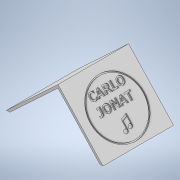
# Autodesk Inventor part: Tableros
Saved by Autodesk Inventor 2022.5 (Build 265521000, 521)
## iProperties
Created: 2023-09-03
Part Number: Tableros
Material: Genérico
Document SubType Name: Modeling
Designer: Carlos_Caucali
Density: 1 g/cm^3
Appearance: Valor por defecto
Author: Carlos_Caucali
Autodesk Inventor part; units mm, degrees
ref_plane "YZ Plane" through (0, 0, 0) normal (1, 0, 0) x (0, 1, 0)
ref_plane "XZ Plane" through (0, 0, 0) normal (0, 1, 0) x (-1, 0, 0)
ref_plane "XY Plane" through (0, 0, 0) normal (0, 0, 1) x (1, 0, 0)
sketch "Boceto1" plane through (0, 0, 0) normal (0, 0, 1) x (1, 0, 0)
  line L0 (0, 204.6955) -> (191.0491, 0) construction
  line L1 (191.0491, 0) -> (183.7386, -6.8232) construction
  line L2 (183.7386, -6.8232) -> (-7.3106, 197.8723) construction
  line L3 (-7.3106, 197.8723) -> (0, 204.6955)
  line L4 (0, 204.6955) -> (-219.3166, 0) construction
  line L5 (-219.3166, 0) -> (-212.4934, -7.3106) construction
  line L6 (-212.4934, -7.3106) -> (6.8232, 197.3849) construction
  line L7 (6.8232, 197.3849) -> (0, 204.6955)
  line L8 (0, 0) -> (0, 350) construction
  line L9 (-300, 0) -> (300, 0) construction
  line L10 (6.8232, 197.3849) -> (191.0491, 0)
  line L11 (177.3703, 0) -> (191.0491, 0)
  line L12 (0, 191.0166) -> (177.3703, 0)
  arc A0 (0, 191.0166) -> (-204.6607, 0) centre (37241.4186, -39915.6513) ccw
  line L13 (-204.6607, 0) -> (-219.3166, 0)
  line L14 (-204.6607, 0) -> (-219.3166, 0)
  line L15 (-219.3166, 0) -> (-7.3106, 197.8723)
  dimension "d0" = 280
  dimension "d1" = 300
  dimension "d2" = 10
  dimension "d3" = 10
  dimension "d4" = 350
  dimension "d5" = 600
  dimension "d6" = 0
  constraints: 30 end point, 7 point on line, 4 parallel, 2 horizontal, 2 perpendicular, 2 point on circle, 1 centre point, 1 collinear, 1 vertical, 10 other
  measures "d0" distance between parallel lines of L1 L4
  measures "d1" distance between parallel lines of L0 L5
  measures "d2" distance between parallel lines of L0 L2
  measures "d3" distance between parallel lines of L6 L4
  measures "d4" distance of L8.start L8.end
  measures "d5" distance of point (-300, 0) point (300, 0)
  measures "d6" distance of L8.start point (0, 0)
extrude "Extrusión1" add sketch "Boceto1" along normal mid plane 300
sketch "Boceto2" plane through (0, 204.6955, 150) normal (0.7310553, 0.6823183, 0) x (0, 0, -1)
  line L0 (300, 0) -> (0, 0) construction
  line L1 (0, -280) -> (0, 0) construction
  line L2 (300, -280) -> (0, -280) construction
  line L3 (300, 0) -> (300, -280) construction
  line L4 (60, -69.6437) -> (240, -69.6437) construction
  line L5 (240, -69.6437) -> (240, -229.6437) construction
  line L6 (240, -229.6437) -> (60, -229.6437) construction
  line L7 (60, -229.6437) -> (60, -69.6437) construction
  circle A0 centre (150, -149.6437) radius 110
  line L8 (60, -69.6437) -> (240, -229.6437) construction
  line L9 (60, -229.6437) -> (240, -69.6437) construction
  circle A1 centre (150, -149.6437) radius 115
  spline S0 degree 2 poles (91.8476, -100.4233) (84.6386, -100.4233) (76.1848, -91.7102) (76.1848, -83.8269) knots 0 0 0 1 2 2 2
  spline S1 degree 2 poles (76.1848, -83.8269) (76.1848, -76.2288) (84.6645, -67.1786) (91.8736, -67.1786) knots 0 0 0 1 2 2 2
  spline S2 degree 2 poles (91.8736, -67.1786) (93.7666, -67.1786) (96.8266, -67.6194) (98.2269, -67.9825) knots 0 0 0 1 2 2 2
  spline S3 degree 2 poles (98.2269, -67.9825) (99.316, -68.3196) (101.8833, -69.4347) (102.6872, -69.8496) knots 0 0 0 1 2 2 2
  line L10 (102.6872, -69.8496) -> (102.6872, -77.4736)
  line L11 (102.6872, -77.4736) -> (101.8833, -77.4736)
  spline S4 degree 2 poles (101.8833, -77.4736) (101.2869, -76.9549) (99.5235, -75.5027) (98.4084, -74.8285) knots 0 0 0 1 2 2 2
  spline S5 degree 2 poles (98.4084, -74.8285) (97.2934, -74.1284) (94.6224, -73.1689) (93.1442, -73.1689) knots 0 0 0 1 2 2 2
  spline S6 degree 2 poles (93.1442, -73.1689) (91.4068, -73.1689) (88.5284, -74.258) (87.2058, -75.6324) knots 0 0 0 1 2 2 2
  spline S7 degree 2 poles (87.2058, -75.6324) (86.013, -76.8512) (84.483, -81.0262) (84.483, -83.8528) knots 0 0 0 1 2 2 2
  spline S8 degree 2 poles (84.483, -83.8528) (84.483, -86.835) (86.0648, -90.9063) (87.3614, -92.151) knots 0 0 0 1 2 2 2
  spline S9 degree 2 poles (87.3614, -92.151) (88.6062, -93.3698) (91.6661, -94.4331) (93.1961, -94.4331) knots 0 0 0 1 2 2 2
  spline S10 degree 2 poles (93.1961, -94.4331) (94.778, -94.4331) (97.6564, -93.3698) (98.6418, -92.7215) knots 0 0 0 1 2 2 2
  spline S11 degree 2 poles (98.6418, -92.7215) (99.731, -92.0733) (101.3647, -90.6989) (101.9611, -90.1543) knots 0 0 0 1 2 2 2
  line L12 (101.9611, -90.1543) -> (102.6872, -90.1543)
  line L13 (102.6872, -90.1543) -> (102.6872, -97.6745)
  spline S12 degree 2 poles (102.6872, -97.6745) (101.8055, -98.0895) (99.4976, -99.1267) (98.2528, -99.4898) knots 0 0 0 1 2 2 2
  spline S13 degree 2 poles (98.2528, -99.4898) (96.7488, -99.9566) (94.1297, -100.4233) (91.8476, -100.4233) knots 0 0 0 1 2 2 2
  line L14 (103.9838, -99.801) -> (114.7974, -67.801)
  line L15 (114.7974, -67.801) -> (123.5624, -67.801)
  line L16 (123.5624, -67.801) -> (134.376, -99.801)
  line L17 (134.376, -99.801) -> (126.1037, -99.801)
  line L18 (126.1037, -99.801) -> (124.107, -93.2661)
  line L19 (124.107, -93.2661) -> (114.0454, -93.2661)
  line L20 (114.0454, -93.2661) -> (112.0227, -99.801)
  line L21 (112.0227, -99.801) -> (103.9838, -99.801)
  line L22 (122.3436, -87.4574) -> (119.0762, -76.8771)
  line L23 (119.0762, -76.8771) -> (115.7828, -87.4574)
  line L24 (115.7828, -87.4574) -> (122.3436, -87.4574)
  line L25 (167.128, -99.801) -> (157.3517, -99.801)
  line L26 (157.3517, -99.801) -> (148.457, -88.0538)
  line L27 (148.457, -88.0538) -> (145.5527, -88.0538)
  line L28 (145.5527, -88.0538) -> (145.5527, -99.801)
  line L29 (145.5527, -99.801) -> (137.5656, -99.801)
  line L30 (137.5656, -99.801) -> (137.5656, -67.801)
  line L31 (137.5656, -67.801) -> (150.4279, -67.801)
  spline S14 degree 2 poles (150.4279, -67.801) (153.0989, -67.801) (157.0405, -68.4752) (158.7261, -69.5125) knots 0 0 0 1 2 2 2
  spline S15 degree 2 poles (158.7261, -69.5125) (160.4376, -70.6016) (162.4603, -73.9987) (162.4603, -76.5919) knots 0 0 0 1 2 2 2
  spline S16 degree 2 poles (162.4603, -76.5919) (162.4603, -80.2483) (159.141, -84.8382) (156.3663, -86.1867) knots 0 0 0 1 2 2 2
  line L32 (156.3663, -86.1867) -> (167.128, -99.801)
  spline S17 degree 2 poles (154.2139, -77.6032) (154.2139, -76.3844) (153.2804, -74.647) (152.2172, -74.1802) knots 0 0 0 1 2 2 2
  spline S18 degree 2 poles (152.2172, -74.1802) (151.4652, -73.869) (149.624, -73.6875) (148.2496, -73.6875) knots 0 0 0 1 2 2 2
  line L33 (148.2496, -73.6875) -> (145.5527, -73.6875)
  line L34 (145.5527, -73.6875) -> (145.5527, -82.2969)
  line L35 (145.5527, -82.2969) -> (147.8606, -82.2969)
  spline S19 degree 2 poles (147.8606, -82.2969) (149.5203, -82.2969) (151.8801, -81.882) (152.684, -81.2337) knots 0 0 0 1 2 2 2
  spline S20 degree 2 poles (152.684, -81.2337) (153.4619, -80.6113) (154.2139, -78.9517) (154.2139, -77.6032) knots 0 0 0 1 2 2 2
  line L36 (190.8558, -99.801) -> (169.5138, -99.801)
  line L37 (169.5138, -99.801) -> (169.5138, -67.801)
  line L38 (169.5138, -67.801) -> (177.5527, -67.801)
  line L39 (177.5527, -67.801) -> (177.5527, -93.707)
  line L40 (177.5527, -93.707) -> (190.8558, -93.707)
  line L41 (190.8558, -93.707) -> (190.8558, -99.801)
  spline S21 degree 2 poles (223.8152, -83.801) (223.8152, -91.5805) (215.517, -100.4752) (208.3079, -100.4752) knots 0 0 0 1 2 2 2
  spline S22 degree 2 poles (208.3079, -100.4752) (201.0729, -100.4752) (192.8266, -91.4768) (192.8266, -83.801) knots 0 0 0 1 2 2 2
  spline S23 degree 2 poles (192.8266, -83.801) (192.8266, -76.0992) (201.0729, -67.1267) (208.3079, -67.1267) knots 0 0 0 1 2 2 2
  spline S24 degree 2 poles (208.3079, -67.1267) (215.517, -67.1267) (223.8152, -76.0473) (223.8152, -83.801) knots 0 0 0 1 2 2 2
  spline S25 degree 2 poles (215.517, -83.801) (215.517, -80.9225) (214.3501, -76.9031) (213.3387, -75.6324) knots 0 0 0 1 2 2 2
  spline S26 degree 2 poles (213.3387, -75.6324) (212.3274, -74.3099) (209.7342, -73.1689) (208.3339, -73.1689) knots 0 0 0 1 2 2 2
  spline S27 degree 2 poles (208.3339, -73.1689) (206.8558, -73.1689) (204.4441, -74.2321) (203.329, -75.5805) knots 0 0 0 1 2 2 2
  spline S28 degree 2 poles (203.329, -75.5805) (202.3436, -76.8253) (201.1248, -80.9485) (201.1248, -83.801) knots 0 0 0 1 2 2 2
  spline S29 degree 2 poles (201.1248, -83.801) (201.1248, -86.7572) (202.2917, -90.647) (203.3031, -91.9695) knots 0 0 0 1 2 2 2
  spline S30 degree 2 poles (203.3031, -91.9695) (204.3144, -93.2921) (206.9335, -94.4331) (208.3339, -94.4331) knots 0 0 0 1 2 2 2
  spline S31 degree 2 poles (208.3339, -94.4331) (209.7601, -94.4331) (212.4052, -93.2143) (213.3647, -91.9177) knots 0 0 0 1 2 2 2
  spline S32 degree 2 poles (213.3647, -91.9177) (214.4019, -90.5173) (215.517, -86.8091) (215.517, -83.801) knots 0 0 0 1 2 2 2
  spline S33 degree 2 poles (95.6467, -143.1008) (95.6467, -145.1753) (94.2204, -148.8576) (92.7942, -150.1542) knots 0 0 0 1 2 2 2
  spline S34 degree 2 poles (92.7942, -150.1542) (91.1864, -151.6064) (86.8039, -152.9808) (83.9514, -152.9808) knots 0 0 0 1 2 2 2
  spline S35 degree 2 poles (83.9514, -152.9808) (81.825, -152.9808) (78.0908, -152.6696) (76.6645, -152.3585) knots 0 0 0 1 2 2 2
  line L42 (76.6645, -152.3585) -> (76.6645, -145.8755)
  line L43 (76.6645, -145.8755) -> (77.3906, -145.8755)
  spline S36 degree 2 poles (77.3906, -145.8755) (78.3501, -146.2645) (80.4506, -146.9387) (82.1102, -146.9387) knots 0 0 0 1 2 2 2
  spline S37 degree 2 poles (82.1102, -146.9387) (84.2366, -146.9387) (86.5446, -145.7458) (87.0113, -144.6567) knots 0 0 0 1 2 2 2
  spline S38 degree 2 poles (87.0113, -144.6567) (87.504, -143.5935) (87.6078, -140.8447) (87.6078, -139.1332) knots 0 0 0 1 2 2 2
  line L44 (87.6078, -139.1332) -> (87.6078, -126.2969)
  line L45 (87.6078, -126.2969) -> (80.295, -126.2969)
  line L46 (80.295, -126.2969) -> (80.295, -120.4881)
  line L47 (80.295, -120.4881) -> (95.6467, -120.4881)
  line L48 (95.6467, -120.4881) -> (95.6467, -143.1008)
  spline S39 degree 2 poles (130.9919, -136.4881) (130.9919, -144.2677) (122.6937, -153.1623) (115.4846, -153.1623) knots 0 0 0 1 2 2 2
  spline S40 degree 2 poles (115.4846, -153.1623) (108.2496, -153.1623) (100.0032, -144.164) (100.0032, -136.4881) knots 0 0 0 1 2 2 2
  spline S41 degree 2 poles (100.0032, -136.4881) (100.0032, -128.7863) (108.2496, -119.8139) (115.4846, -119.8139) knots 0 0 0 1 2 2 2
  spline S42 degree 2 poles (115.4846, -119.8139) (122.6937, -119.8139) (130.9919, -128.7345) (130.9919, -136.4881) knots 0 0 0 1 2 2 2
  spline S43 degree 2 poles (122.6937, -136.4881) (122.6937, -133.6097) (121.5267, -129.5902) (120.5154, -128.3196) knots 0 0 0 1 2 2 2
  spline S44 degree 2 poles (120.5154, -128.3196) (119.504, -126.997) (116.9109, -125.856) (115.5105, -125.856) knots 0 0 0 1 2 2 2
  spline S45 degree 2 poles (115.5105, -125.856) (114.0324, -125.856) (111.6207, -126.9192) (110.5057, -128.2677) knots 0 0 0 1 2 2 2
  spline S46 degree 2 poles (110.5057, -128.2677) (109.5203, -129.5124) (108.3015, -133.6356) (108.3015, -136.4881) knots 0 0 0 1 2 2 2
  spline S47 degree 2 poles (108.3015, -136.4881) (108.3015, -139.4444) (109.4684, -143.3341) (110.4797, -144.6567) knots 0 0 0 1 2 2 2
  spline S48 degree 2 poles (110.4797, -144.6567) (111.4911, -145.9792) (114.1102, -147.1202) (115.5105, -147.1202) knots 0 0 0 1 2 2 2
  spline S49 degree 2 poles (115.5105, -147.1202) (116.9368, -147.1202) (119.5818, -145.9014) (120.5413, -144.6048) knots 0 0 0 1 2 2 2
  spline S50 degree 2 poles (120.5413, -144.6048) (121.5786, -143.2045) (122.6937, -139.4962) (122.6937, -136.4881) knots 0 0 0 1 2 2 2
  line L49 (163.1734, -152.4881) -> (155.4457, -152.4881)
  line L50 (155.4457, -152.4881) -> (143.1021, -130.1867)
  line L51 (143.1021, -130.1867) -> (143.1021, -152.4881)
  line L52 (143.1021, -152.4881) -> (135.7634, -152.4881)
  line L53 (135.7634, -152.4881) -> (135.7634, -120.4881)
  line L54 (135.7634, -120.4881) -> (145.6175, -120.4881)
  line L55 (145.6175, -120.4881) -> (155.8347, -138.822)
  line L56 (155.8347, -138.822) -> (155.8347, -120.4881)
  line L57 (155.8347, -120.4881) -> (163.1734, -120.4881)
  line L58 (163.1734, -120.4881) -> (163.1734, -152.4881)
  line L59 (166.2334, -152.4881) -> (177.047, -120.4881)
  line L60 (177.047, -120.4881) -> (185.812, -120.4881)
  line L61 (185.812, -120.4881) -> (196.6256, -152.4881)
  line L62 (196.6256, -152.4881) -> (188.3533, -152.4881)
  line L63 (188.3533, -152.4881) -> (186.3566, -145.9533)
  line L64 (186.3566, -145.9533) -> (176.295, -145.9533)
  line L65 (176.295, -145.9533) -> (174.2723, -152.4881)
  line L66 (174.2723, -152.4881) -> (166.2334, -152.4881)
  line L67 (184.5932, -140.1445) -> (181.3258, -129.5643)
  line L68 (181.3258, -129.5643) -> (178.0324, -140.1445)
  line L69 (178.0324, -140.1445) -> (184.5932, -140.1445)
  line L70 (205.9611, -152.4881) -> (205.9611, -126.5821)
  line L71 (205.9611, -126.5821) -> (196.4959, -126.5821)
  line L72 (196.4959, -126.5821) -> (196.4959, -120.4881)
  line L73 (196.4959, -120.4881) -> (223.4652, -120.4881)
  line L74 (223.4652, -120.4881) -> (223.4652, -126.5821)
  line L75 (223.4652, -126.5821) -> (214, -126.5821)
  line L76 (214, -126.5821) -> (214, -152.4881)
  line L77 (214, -152.4881) -> (205.9611, -152.4881)
  line L78 (142.1191, -185.1591) -> (168.8614, -176.8527)
  line L79 (168.8614, -176.8527) -> (168.8614, -214.0488)
  spline S51 degree 2 poles (168.8614, -214.0488) (168.8614, -218.2223) (166.7545, -222.4362) (161.6896, -225.1915) (158.4887, -225.1915) knots 0 0 0 1 2 3 3 3
  spline S52 degree 2 poles (158.4887, -225.1915) (154.842, -225.1915) (150.466, -220.9775) (150.466, -217.655) knots 0 0 0 1 2 2 2
  spline S53 degree 2 poles (150.466, -217.655) (150.466, -214.292) (155.6524, -209.4297) (159.7447, -209.4297) knots 0 0 0 1 2 2 2
  spline S54 degree 2 poles (159.7447, -209.4297) (161.0818, -209.4297) (163.1078, -209.9159) (165.4579, -210.8884) knots 0 0 0 1 2 2 2
  line L80 (165.4579, -210.8884) -> (165.4579, -186.5772)
  line L81 (165.4579, -186.5772) -> (145.4822, -192.7766)
  line L82 (145.4822, -192.7766) -> (145.4822, -220.856)
  spline S55 degree 2 poles (145.4822, -220.856) (145.4822, -224.9484) (143.2942, -229.4864) (138.0673, -232.1607) (134.9878, -232.1607) knots 0 0 0 1 2 3 3 3
  spline S56 degree 2 poles (134.9878, -232.1607) (131.3412, -232.1607) (127.0462, -228.0278) (127.0462, -224.7052) knots 0 0 0 1 2 2 2
  spline S57 degree 2 poles (127.0462, -224.7052) (127.0462, -221.1801) (132.1515, -216.3989) (136.2844, -216.3989) knots 0 0 0 1 2 2 2
  spline S58 degree 2 poles (136.2844, -216.3989) (138.9182, -216.3989) (142.1191, -217.9386) knots 0 0 0 1 1 1
  line L83 (142.1191, -217.9386) -> (142.1191, -185.1591)
  dimension "d9" = 220
  dimension "d10" = 180
  dimension "d11" = 160
  dimension "d12" = 230
  constraints: 4 end point, 3 coincident, 2 centre point, 1 midpoint, 2 other
  measures "d9" diameter of A0
  measures "d10" distance of L4.start L4.end
  measures "d11" distance of L6.end L4.start
  measures "d12" diameter of A1
extrude "Extrusión2" cut sketch "Boceto2" against normal blind 5
equation "\"d3\" = d2"
